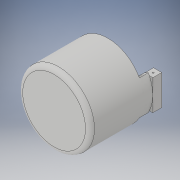
# Autodesk Inventor part: ballcarriage
Saved by Autodesk Inventor 2018 (Build 220112000, 112)
## iProperties
Created: 2019-05-07
Part Number: ballcarriage
Material: Generic
Document SubType Name: Modeling
Designer: F8PLTW
Density: 1 g/cm^3
Appearance: Default
Author: F8PLTW
Autodesk Inventor part; units mm, degrees
ref_plane "YZ Plane" through (0, 0, 0) normal (1, 0, 0) x (0, 1, 0)
ref_plane "XZ Plane" through (0, 0, 0) normal (0, 1, 0) x (-1, 0, 0)
ref_plane "XY Plane" through (0, 0, 0) normal (0, 0, 1) x (1, 0, 0)
sketch "Sketch1" plane through (0, 0, 0) normal (0, 0, 1) x (1, 0, 0)
  circle A0 centre (-4.4309, 2.4544) radius 22.335
  circle A1 centre (-4.4309, 2.4544) radius 25.4
  point P0 (0, 0)
  dimension "d0" = 44.67
  dimension "d1" = 50.8
  constraints: 2 centre point, 1 coincident
  measures "d0" diameter of A0
  measures "d1" diameter of A1
extrude "Extrusion1" add sketch "Sketch1" along normal blind 25.4
sketch "Sketch2" plane through (-4.4309, 2.4544, 25.4) normal (0, 0, 1) x (1, 0, 0)
  circle A0 centre (0, 0) radius 25.4
  point P0 (4.4309, -2.4544)
  constraints: 1 centre point
extrude "Extrusion2" add sketch "Sketch2" along normal blind 12.7
fillet "Fillet1" radius 3.175 1 edges at (-29.8309, 2.4544, 38.1)
sketch "Sketch3" plane through (-4.4309, 2.4544, 0) normal (0, 0, -1) x (-1, 0, 0)
  circle A0 centre (0, 0) radius 25.4 projected
  arc A1 (-22.2614, 12.2307) -> (-22.2614, -12.2307) centre (0, 0) ccw
  line L0 (-22.2614, 12.2307) -> (-22.2614, -12.2307) construction
  line L1 (-22.2614, 12.2307) -> (2.1999, 12.2307) construction
  circle A2 centre (0, 0) radius 22.225 projected
  arc A3 (-19.4415, 10.7694) -> (-19.4415, -10.7694) centre (0, 0) ccw
  line L2 (-19.4415, 10.7694) -> (-19.4415, -10.7694) construction
  line L3 (-19.4415, 10.7694) -> (2.0972, 10.7694) construction
  line L4 (-22.2614, -12.2307) -> (-19.4415, -10.7694)
  line L5 (-22.2614, 12.2307) -> (-19.4415, 10.7694)
  point P0 (-4.4309, -2.4544)
  dimension "d7" = 90
  dimension "d8" = 90
  constraints: 12 end point, 8 point on circle, 2 centre point, 2 horizontal, 2 perpendicular
  measures "d7" angle of L0 L1
  measures "d8" angle of L2 L3
extrude "Extrusion3" add sketch "Sketch3" along normal blind 6.35 contours L5 A2 L4 A0 picked at (-24.2184, -0.7482)
sketch "Sketch4" plane through (-4.4309, 2.4544, -6.35) normal (0, 0, -1) x (-1, 0, 0)
  circle A0 centre (0, 0) radius 22.335 projected
  line L0 (-19.5898, 10.728) -> (-25.4, 10.728)
  line L1 (-25.4, 10.728) -> (-25.4, -10.7831)
  line L2 (-25.4, -10.7831) -> (-19.5898, -10.7831)
  line L3 (-19.5898, -10.7831) -> (-19.5898, 10.728)
  point P0 (-4.4309, -2.4544)
  constraints: 8 end point, 2 parallel, 1 horizontal, 1 perpendicular, 2 other
extrude "Extrusion4" add sketch "Sketch4" along normal blind 6.35 contours L3 A0 | A0 L3 L2 L1 L0 picked at (-20.171, -2.2046)
sketch "Sketch5" plane through (-4.4309, 2.4544, -6.35) normal (0, 0, -1) x (-1, 0, 0)
  point P0 (-4.4309, -2.4544)
sketch "Sketch6" plane through (18.5665, -8.3288, -6.35) normal (0, -1, 0) x (1, 0, 0)
  line L0 (-3.4076, -6.35) -> (2.4025, -6.35) projected
  line L1 (-3.4076, 0) -> (0, 0) projected
  line L2 (2.4025, -6.35) -> (-3.4076, 0) construction
  line L3 (-3.4076, -6.35) -> (2.4025, 0) construction
  line L4 (2.4025, 0) -> (2.4025, 41.275) projected
  circle A0 centre (-0.5026, -3.175) radius 0.5
  point P0 (-18.5665, 6.35)
  dimension "d13" = 1
  constraints: 4 end point, 1 centre point, 1 midpoint, 1 point on line
  measures "d13" diameter of A0
extrude "Extrusion5" cut sketch "Sketch6" against normal blind 25.4
body "Solid1"
